Autodesk Inventor part; units mm, degrees
(part 4 of 4)
  arc A427 (4.3874, -10.8619) -> (4.7253, -10.6897) centre (-4.2393, 6.4866) ccw
  arc A428 (4.7253, -10.6897) -> (4.9404, -10.9173) centre (8.6621, -7.1833) ccw
  arc A429 (4.9404, -10.9173) -> (5.2279, -11.1867) centre (9.4643, -6.3793) ccw
  arc A430 (5.2279, -11.1867) -> (5.6027, -11.4963) centre (10.2445, -5.4945) ccw
  arc A431 (5.6027, -11.4963) -> (5.9512, -11.3011) centre (-4.2393, 6.4866) ccw
  arc A432 (5.9512, -11.3011) -> (5.8831, -10.8198) centre (-1.5915, -12.123) ccw
  arc A433 (5.8831, -10.8198) -> (5.8036, -10.4339) centre (-0.4294, -11.92) ccw
  arc A434 (5.8036, -10.4339) -> (5.7219, -10.1316) centre (0.6753, -11.6561) ccw
  arc A435 (5.7219, -10.1316) -> (6.0453, -9.9334) centre (-4.2393, 6.4866) ccw
  arc A436 (6.0453, -9.9334) -> (6.2776, -10.1434) centre (9.6948, -6.1289) ccw
  arc A437 (6.2776, -10.1434) -> (6.5853, -10.3895) centre (10.4315, -5.2644) ccw
  arc A438 (6.5853, -10.3895) -> (6.9833, -10.6687) centre (11.1399, -4.3212) ccw
  arc A439 (6.9833, -10.6687) -> (7.3154, -10.4467) centre (-4.2393, 6.4866) ccw
  arc A440 (7.3154, -10.4467) -> (7.2097, -9.9722) centre (-0.1395, -11.8579) ccw
  arc A441 (7.2097, -9.9722) -> (7.1002, -9.5938) centre (1.003, -11.5644) ccw
  arc A442 (7.1002, -9.5938) -> (6.9951, -9.2988) centre (2.0836, -11.2146) ccw
  arc A443 (6.9951, -9.2988) -> (7.3019, -9.0759) centre (-4.2393, 6.4866) ccw
  arc A444 (7.3019, -9.0759) -> (7.55, -9.267) centre (10.6417, -4.9968) ccw
  arc A445 (7.55, -9.267) -> (7.876, -9.4881) centre (11.3083, -4.0772) ccw
  arc A446 (7.876, -9.4881) -> (8.2947, -9.7353) centre (11.9405, -3.0813) ccw
  arc A447 (8.2947, -9.7353) -> (8.6084, -9.488) centre (-4.2393, 6.4866) ccw
  arc A448 (8.6084, -9.488) -> (8.4658, -9.0232) centre (1.2871, -11.4797) ccw
  arc A449 (8.4658, -9.0232) -> (8.3269, -8.6545) centre (2.4031, -11.0974) ccw
  arc A450 (8.3269, -8.6545) -> (8.199, -8.3687) centre (3.4529, -10.664) ccw
  arc A451 (8.199, -8.3687) -> (8.4873, -8.1224) centre (-4.2393, 6.4866) ccw
  arc A452 (8.4873, -8.1224) -> (8.7497, -8.2934) centre (11.4968, -3.7938) ccw
  arc A453 (8.7497, -8.2934) -> (9.0921, -8.4883) centre (12.0892, -2.8247) ccw
  arc A454 (9.0921, -8.4883) -> (9.5288, -8.7019) centre (12.6413, -1.7823) ccw
  arc A455 (9.5288, -8.7019) -> (9.8221, -8.4307) centre (-4.2393, 6.4866) ccw
  arc A456 (9.8221, -8.4307) -> (9.6435, -7.9786) centre (2.6797, -10.9907) ccw
  arc A457 (9.6435, -7.9786) -> (9.4761, -7.6219) centre (3.7622, -10.5221) ccw
  arc A458 (9.4761, -7.6219) -> (9.3261, -7.347) centre (4.7748, -10.0076) ccw
  arc A459 (9.3261, -7.347) -> (9.5943, -7.0788) centre (-4.2393, 6.4866) ccw
  arc A460 (9.5943, -7.0788) -> (9.8693, -7.2288) centre (12.2549, -2.5275) ccw
  arc A461 (9.8693, -7.2288) -> (10.2259, -7.3962) centre (12.7694, -1.5149) ccw
  arc A462 (10.2259, -7.3962) -> (10.678, -7.5748) centre (13.238, -0.4324) ccw
  arc A463 (10.678, -7.5748) -> (10.9492, -7.2815) centre (-4.2393, 6.4866) ccw
  arc A464 (10.9492, -7.2815) -> (10.7357, -6.8447) centre (4.0296, -10.394) ccw
  arc A465 (10.7357, -6.8447) -> (10.5408, -6.5023) centre (5.0721, -9.8418) ccw
  arc A466 (10.5408, -6.5023) -> (10.3697, -6.24) centre (6.0411, -9.2495) ccw
  arc A467 (10.3697, -6.24) -> (10.616, -5.9516) centre (-4.2393, 6.4866) ccw
  arc A468 (10.616, -5.9516) -> (10.9019, -6.0795) centre (12.9113, -1.2056) ccw
  arc A469 (10.9019, -6.0795) -> (11.2705, -6.2185) centre (13.3447, -0.1558) ccw
  arc A470 (11.2705, -6.2185) -> (11.7353, -6.3611) centre (13.727, 0.9602) ccw
  arc A471 (11.7353, -6.3611) -> (11.9826, -6.0473) centre (-4.2393, 6.4866) ccw
  arc A472 (11.9826, -6.0473) -> (11.7355, -5.6287) centre (5.3286, -9.6932) ccw
  arc A473 (11.7355, -5.6287) -> (11.5143, -5.3027) centre (6.3245, -9.0609) ccw
  arc A474 (11.5143, -5.3027) -> (11.3232, -5.0546) centre (7.2441, -8.3944) ccw
  arc A475 (11.3232, -5.0546) -> (11.5461, -4.7478) centre (-4.2393, 6.4866) ccw
  arc A476 (11.5461, -4.7478) -> (11.8411, -4.8528) centre (13.4619, 0.1637) ccw
  arc A477 (11.8411, -4.8528) -> (12.2196, -4.9624) centre (13.8117, 1.2443) ccw
  arc A478 (12.2196, -4.9624) -> (12.694, -5.0681) centre (14.1052, 2.3868) ccw
  arc A479 (12.694, -5.0681) -> (12.916, -4.736) centre (-4.2393, 6.4866) ccw
  arc A480 (12.916, -4.736) -> (12.6368, -4.338) centre (6.5685, -8.8926) ccw
  arc A481 (12.6368, -4.338) -> (12.3907, -4.0303) centre (7.5118, -8.1842) ccw
  arc A482 (12.3907, -4.0303) -> (12.1807, -3.798) centre (8.3762, -7.4475) ccw
  arc A483 (12.1807, -3.798) -> (12.3789, -3.4746) centre (-4.2393, 6.4866) ccw
  arc A484 (12.3789, -3.4746) -> (12.6812, -3.5562) centre (13.9035, 1.5721) ccw
  arc A485 (12.6812, -3.5562) -> (13.0671, -3.6358) centre (14.1674, 2.6768) ccw
  arc A486 (13.0671, -3.6358) -> (13.5484, -3.7039) centre (14.3703, 3.8388) ccw
  arc A487 (13.5484, -3.7039) -> (13.7436, -3.3554) centre (-4.2393, 6.4866) ccw
  arc A488 (13.7436, -3.3554) -> (13.434, -2.9806) centre (7.7419, -7.9972) ccw
  arc A489 (13.434, -2.9806) -> (13.1646, -2.6931) centre (8.6266, -7.217) ccw
  arc A490 (13.1646, -2.6931) -> (12.937, -2.478) centre (9.4306, -6.4148) ccw
  arc A491 (12.937, -2.478) -> (13.1092, -2.1401) centre (-4.2393, 6.4866) ccw
  arc A492 (13.1092, -2.1401) -> (13.417, -2.1977) centre (14.2331, 3.0107) ccw
  arc A493 (13.417, -2.1977) -> (13.8079, -2.2467) centre (14.4095, 4.1327) ccw
  arc A494 (13.8079, -2.2467) -> (14.2931, -2.2769) centre (14.5207, 5.307) ccw
  arc A495 (14.2931, -2.2769) -> (14.4604, -1.9141) centre (-4.2393, 6.4866) ccw
  arc A496 (14.4604, -1.9141) -> (14.1223, -1.5647) centre (8.8413, -7.0125) ccw
  arc A497 (14.1223, -1.5647) -> (13.8312, -1.2993) centre (9.6621, -6.1653) ccw
  arc A498 (13.8312, -1.2993) -> (13.5874, -1.1027) centre (10.4007, -5.3025) ccw
  arc A499 (13.5874, -1.1027) -> (13.7326, -0.7523) centre (-4.2393, 6.4866) ccw
  arc A500 (13.7326, -0.7523) -> (14.044, -0.7856) centre (14.4489, 4.4707) ccw
  arc A501 (14.044, -0.7856) -> (14.4375, -0.8038) centre (14.5367, 5.6031) ccw
  arc A502 (14.4375, -0.8038) -> (14.9236, -0.7958) centre (14.5554, 6.7826) ccw
  arc A503 (14.9236, -0.7958) -> (15.0618, -0.4211) centre (-4.2393, 6.4866) ccw
  arc A504 (15.0618, -0.4211) -> (14.6974, -0.0993) centre (9.8601, -5.9446) ccw
  arc A505 (14.6974, -0.0993) -> (14.3864, 0.1425) centre (10.6119, -5.0356) ccw
  arc A506 (14.3864, 0.1425) -> (14.1279, 0.3194) centre (11.2805, -4.1175) ccw
  arc A507 (14.1279, 0.3194) -> (14.2451, 0.6801) centre (-4.2393, 6.4866) ccw
  arc A508 (14.2451, 0.6801) -> (14.5582, 0.6713) centre (14.5494, 5.9432) ccw
  arc A509 (14.5582, 0.6713) -> (14.9519, 0.684) centre (14.5482, 7.079) ccw
  arc A510 (14.9519, 0.684) -> (15.4359, 0.7301) centre (14.4743, 8.2563) ccw
  arc A511 (15.4359, 0.7301) -> (15.5443, 1.1146) centre (-4.2393, 6.4866) ccw
  arc A512 (15.5443, 1.1146) -> (15.1558, 1.4068) centre (10.792, -4.8001) ccw
  arc A513 (15.1558, 1.4068) -> (14.8267, 1.6234) centre (11.4701, -3.8349) ccw
  arc A514 (14.8267, 1.6234) -> (14.5552, 1.7794) centre (12.0647, -2.8671) ccw
  arc A515 (14.5552, 1.7794) -> (14.6437, 2.1482) centre (-4.2393, 6.4866) ccw
  arc A516 (14.6437, 2.1482) -> (14.9565, 2.164) centre (14.5342, 7.419) ccw
  arc A517 (14.9565, 2.164) -> (15.3481, 2.2076) centre (14.4438, 8.5512) ccw
  arc A518 (15.3481, 2.2076) -> (15.8269, 2.2916) centre (14.2777, 9.7191) ccw
  arc A519 (15.8269, 2.2916) -> (15.9048, 2.6834) centre (-4.2393, 6.4866) ccw
  arc A520 (15.9048, 2.6834) -> (15.4946, 2.9442) centre (11.6312, -3.5859) ccw
  arc A521 (15.4946, 2.9442) -> (15.1495, 3.1343) centre (12.2315, -2.5705) ccw
  arc A522 (15.1495, 3.1343) -> (14.8666, 3.2686) centre (12.7483, -1.5591) ccw
  arc A523 (14.8666, 3.2686) -> (14.9259, 3.6431) centre (-4.2393, 6.4866) ccw
  arc A524 (14.9259, 3.6431) -> (15.2365, 3.6834) centre (14.4031, 8.8891) ccw
  arc A525 (15.2365, 3.6834) -> (15.6234, 3.7576) centre (14.2242, 10.0107) ccw
  arc A526 (15.6234, 3.7576) -> (16.0942, 3.8789) centre (13.967, 11.1619) ccw
  arc A527 (16.0942, 3.8789) -> (16.1411, 4.2756) centre (-4.2393, 6.4866) ccw
  arc A528 (16.1411, 4.2756) -> (15.7117, 4.5034) centre (12.3726, -2.3097) ccw
  arc A529 (15.7117, 4.5034) -> (15.3527, 4.6658) centre (12.8914, -1.2503) ccw
  arc A530 (15.3527, 4.6658) -> (15.0602, 4.7775) centre (13.3272, -0.2015) ccw
  arc A531 (15.0602, 4.7775) -> (15.0899, 5.1556) centre (-4.2393, 6.4866) ccw
  arc A532 (15.0899, 5.1556) -> (15.3964, 5.2201) centre (14.1572, 10.3443) ccw
  arc A533 (15.3964, 5.2201) -> (15.7763, 5.3244) centre (13.8908, 11.4485) ccw
  arc A534 (15.7763, 5.3244) -> (16.2361, 5.4823) centre (13.5441, 12.576) ccw
  arc A535 (16.2361, 5.4823) -> (16.2518, 5.8814) centre (-4.2393, 6.4866) ccw
  arc A536 (16.2518, 5.8814) -> (15.8058, 6.0748) centre (13.0115, -0.9792) ccw
  arc A537 (15.8058, 6.0748) -> (15.4352, 6.2086) centre (13.4456, 0.1176) ccw
  arc A538 (15.4352, 6.2086) -> (15.1348, 6.297) centre (13.7978, 1.1974) ccw
  arc A539 (15.1348, 6.297) -> (15.1348, 6.6762) centre (-4.2393, 6.4866) ccw
  arc A540 (15.1348, 6.6762) -> (15.4352, 6.7646) centre (13.7978, 11.7758) ccw
  arc A541 (15.4352, 6.7646) -> (15.8058, 6.8984) centre (13.4456, 12.8556) ccw
  arc A542 (15.8058, 6.8984) -> (16.2518, 7.0918) centre (13.0115, 13.9525) ccw
  arc A543 (16.2518, 7.0918) -> (16.2361, 7.491) centre (-4.2393, 6.4866) ccw
  arc A544 (16.2361, 7.491) -> (15.7763, 7.6488) centre (13.5441, 0.3973) ccw
  arc A545 (15.7763, 7.6488) -> (15.3964, 7.7531) centre (13.8908, 1.5248) ccw
  arc A546 (15.3964, 7.7531) -> (15.0899, 7.8177) centre (14.1572, 2.6289) ccw
  arc A547 (15.0899, 7.8177) -> (15.0602, 8.1957) centre (-4.2393, 6.4866) ccw
  arc A548 (15.0602, 8.1957) -> (15.3527, 8.3074) centre (13.3272, 13.1747) ccw
  arc A549 (15.3527, 8.3074) -> (15.7117, 8.4699) centre (12.8914, 14.2235) ccw
  arc A550 (15.7117, 8.4699) -> (16.1411, 8.6977) centre (12.3726, 15.2829) ccw
  arc A551 (16.1411, 8.6977) -> (16.0942, 9.0944) centre (-4.2393, 6.4866) ccw
  arc A552 (16.0942, 9.0944) -> (15.6234, 9.2156) centre (13.967, 1.8113) ccw
  arc A553 (15.6234, 9.2156) -> (15.2365, 9.2898) centre (14.2242, 2.9626) ccw
  arc A554 (15.2365, 9.2898) -> (14.9259, 9.3301) centre (14.4031, 4.0842) ccw
  arc A555 (14.9259, 9.3301) -> (14.8666, 9.7047) centre (-4.2393, 6.4866) ccw
  arc A556 (14.8666, 9.7047) -> (15.1495, 9.839) centre (12.7483, 14.5323) ccw
  arc A557 (15.1495, 9.839) -> (15.4946, 10.0291) centre (12.2315, 15.5438) ccw
  arc A558 (15.4946, 10.0291) -> (15.9048, 10.2899) centre (11.6312, 16.5592) ccw
  arc A559 (15.9048, 10.2899) -> (15.8269, 10.6817) centre (-4.2393, 6.4866) ccw
  arc A560 (15.8269, 10.6817) -> (15.3481, 10.7656) centre (14.2777, 3.2542) ccw
  arc A561 (15.3481, 10.7656) -> (14.9565, 10.8092) centre (14.4438, 4.422) ccw
  arc A562 (14.9565, 10.8092) -> (14.6437, 10.825) centre (14.5342, 5.5542) ccw
  arc A563 (14.6437, 10.825) -> (14.5552, 11.1938) centre (-4.2393, 6.4866) ccw
  arc A564 (14.5552, 11.1938) -> (14.8267, 11.3499) centre (12.0647, 15.8404) ccw
  arc A565 (14.8267, 11.3499) -> (15.1558, 11.5665) centre (11.4701, 16.8081) ccw
  arc A566 (15.1558, 11.5665) -> (15.5443, 11.8587) centre (10.792, 17.7733) ccw
  arc A567 (15.5443, 11.8587) -> (15.4359, 12.2431) centre (-4.2393, 6.4866) ccw
  arc A568 (15.4359, 12.2431) -> (14.9519, 12.2893) centre (14.4743, 4.717) ccw
  arc A569 (14.9519, 12.2893) -> (14.5582, 12.302) centre (14.5482, 5.8943) ccw
  arc A570 (14.5582, 12.302) -> (14.2451, 12.2932) centre (14.5494, 7.0301) ccw
  arc A571 (14.2451, 12.2932) -> (14.1279, 12.6539) centre (-4.2393, 6.4866) ccw
  arc A572 (14.1279, 12.6539) -> (14.3864, 12.8308) centre (11.2805, 17.0907) ccw
  arc A573 (14.3864, 12.8308) -> (14.6974, 13.0725) centre (10.6119, 18.0089) ccw
  arc A574 (14.6974, 13.0725) -> (15.0618, 13.3943) centre (9.8601, 18.9179) ccw
  arc A575 (15.0618, 13.3943) -> (14.9236, 13.7691) centre (-4.2393, 6.4866) ccw
  arc A576 (14.9236, 13.7691) -> (14.4375, 13.7771) centre (14.5554, 6.1907) ccw
  arc A577 (14.4375, 13.7771) -> (14.044, 13.7589) centre (14.5367, 7.3701) ccw
  arc A578 (14.044, 13.7589) -> (13.7326, 13.7256) centre (14.4489, 8.5025) ccw
  arc A579 (13.7326, 13.7256) -> (13.5874, 14.076) centre (-4.2393, 6.4866) ccw
  arc A580 (13.5874, 14.076) -> (13.8312, 14.2726) centre (10.4007, 18.2757) ccw
  arc A581 (13.8312, 14.2726) -> (14.1223, 14.538) centre (9.6621, 19.1385) ccw
  arc A582 (14.1223, 14.538) -> (14.4604, 14.8874) centre (8.8413, 19.9858) ccw
  arc A583 (14.4604, 14.8874) -> (14.2931, 15.2501) centre (-4.2393, 6.4866) ccw
  arc A584 (14.2931, 15.2501) -> (13.8079, 15.22) centre (14.5207, 7.6662) ccw
  arc A585 (13.8079, 15.22) -> (13.417, 15.171) centre (14.4095, 8.8406) ccw
  arc A586 (13.417, 15.171) -> (13.1092, 15.1133) centre (14.2331, 9.9626) ccw
  arc A587 (13.1092, 15.1133) -> (12.937, 15.4512) centre (-4.2393, 6.4866) ccw
  arc A588 (12.937, 15.4512) -> (13.1646, 15.6664) centre (9.4306, 19.388) ccw
  arc A589 (13.1646, 15.6664) -> (13.434, 15.9538) centre (8.6266, 20.1902) ccw
  arc A590 (13.434, 15.9538) -> (13.7436, 16.3286) centre (7.7419, 20.9705) ccw
  arc A591 (13.7436, 16.3286) -> (13.5484, 16.6771) centre (-4.2393, 6.4866) ccw
  arc A592 (13.5484, 16.6771) -> (13.0671, 16.609) centre (14.3703, 9.1345) ccw
  arc A593 (13.0671, 16.609) -> (12.6812, 16.5295) centre (14.1674, 10.2965) ccw
  arc A594 (12.6812, 16.5295) -> (12.3789, 16.4479) centre (13.9035, 11.4012) ccw
  arc A595 (12.3789, 16.4479) -> (12.1807, 16.7712) centre (-4.2393, 6.4866) ccw
  arc A596 (12.1807, 16.7712) -> (12.3907, 17.0036) centre (8.3762, 20.4208) ccw
  arc A597 (12.3907, 17.0036) -> (12.6368, 17.3113) centre (7.5118, 21.1574) ccw
  arc A598 (12.6368, 17.3113) -> (12.916, 17.7092) centre (6.5685, 21.8658) ccw
  arc A599 (12.916, 17.7092) -> (12.694, 18.0413) centre (-4.2393, 6.4866) ccw
  arc A600 (12.694, 18.0413) -> (12.2196, 17.9357) centre (14.1052, 10.5864) ccw
  arc A601 (12.2196, 17.9357) -> (11.8411, 17.8261) centre (13.8117, 11.7289) ccw
  arc A602 (11.8411, 17.8261) -> (11.5461, 17.721) centre (13.4619, 12.8095) ccw
  arc A603 (11.5461, 17.721) -> (11.3232, 18.0278) centre (-4.2393, 6.4866) ccw
  arc A604 (11.3232, 18.0278) -> (11.5143, 18.2759) centre (7.2441, 21.3676) ccw
  arc A605 (11.5143, 18.2759) -> (11.7355, 18.602) centre (6.3245, 22.0342) ccw
  arc A606 (11.7355, 18.602) -> (11.9826, 19.0206) centre (5.3286, 22.6664) ccw
  arc A607 (11.9826, 19.0206) -> (11.7353, 19.3343) centre (-4.2393, 6.4866) ccw
  arc A608 (11.7353, 19.3343) -> (11.2705, 19.1917) centre (13.727, 12.0131) ccw
  arc A609 (11.2705, 19.1917) -> (10.9019, 19.0528) centre (13.3447, 13.129) ccw
  arc A610 (10.9019, 19.0528) -> (10.616, 18.9249) centre (12.9113, 14.1788) ccw
  arc A611 (10.616, 18.9249) -> (10.3697, 19.2133) centre (-4.2393, 6.4866) ccw
  arc A612 (10.3697, 19.2133) -> (10.5408, 19.4756) centre (6.0411, 22.2227) ccw
  arc A613 (10.5408, 19.4756) -> (10.7357, 19.818) centre (5.0721, 22.8151) ccw
  arc A614 (10.7357, 19.818) -> (10.9492, 20.2547) centre (4.0296, 23.3672) ccw
  arc A615 (10.9492, 20.2547) -> (10.678, 20.548) centre (-4.2393, 6.4866) ccw
  arc A616 (10.678, 20.548) -> (10.2259, 20.3695) centre (13.238, 13.4056) ccw
  arc A617 (10.2259, 20.3695) -> (9.8693, 20.202) centre (12.7694, 14.4882) ccw
  arc A618 (9.8693, 20.202) -> (9.5943, 20.0521) centre (12.2549, 15.5007) ccw
  arc A619 (9.5943, 20.0521) -> (9.3261, 20.3202) centre (-4.2393, 6.4866) ccw
  arc A620 (9.3261, 20.3202) -> (9.4761, 20.5952) centre (4.7748, 22.9808) ccw
  arc A621 (9.4761, 20.5952) -> (9.6435, 20.9518) centre (3.7622, 23.4953) ccw
  arc A622 (9.6435, 20.9518) -> (9.8221, 21.4039) centre (2.6797, 23.964) ccw
  arc A623 (9.8221, 21.4039) -> (9.5288, 21.6751) centre (-4.2393, 6.4866) ccw
  arc A624 (9.5288, 21.6751) -> (9.0921, 21.4616) centre (12.6413, 14.7556) ccw
  arc A625 (9.0921, 21.4616) -> (8.7497, 21.2667) centre (12.0892, 15.798) ccw
  arc A626 (8.7497, 21.2667) -> (8.4873, 21.0956) centre (11.4968, 16.7671) ccw
  arc A627 (8.4873, 21.0956) -> (8.199, 21.3419) centre (-4.2393, 6.4866) ccw
  arc A628 (8.199, 21.3419) -> (8.3269, 21.6278) centre (3.4529, 23.6372) ccw
  arc A629 (8.3269, 21.6278) -> (8.4658, 21.9965) centre (2.4031, 24.0707) ccw
  arc A630 (8.4658, 21.9965) -> (8.6084, 22.4612) centre (1.2871, 24.4529) ccw
  arc A631 (8.6084, 22.4612) -> (8.2947, 22.7085) centre (-4.2393, 6.4866) ccw
  arc A632 (8.2947, 22.7085) -> (7.876, 22.4614) centre (11.9405, 16.0545) ccw
  arc A633 (7.876, 22.4614) -> (7.55, 22.2402) centre (11.3083, 17.0504) ccw
  arc A634 (7.55, 22.2402) -> (7.3019, 22.0491) centre (10.6417, 17.97) ccw
  arc A635 (7.3019, 22.0491) -> (6.9951, 22.272) centre (-4.2393, 6.4866) ccw
  arc A636 (6.9951, 22.272) -> (7.1002, 22.567) centre (2.0836, 24.1879) ccw
  arc A637 (7.1002, 22.567) -> (7.2097, 22.9455) centre (1.003, 24.5376) ccw
  arc A638 (7.2097, 22.9455) -> (7.3154, 23.42) centre (-0.1395, 24.8311) ccw
  arc A639 (7.3154, 23.42) -> (6.9833, 23.6419) centre (-4.2393, 6.4866) ccw
  circle A640 centre (-4.2393, 6.4866) radius 2
  circle A641 centre (-4.2393, 6.4866) radius 18.25
  point P0 (0, 0)
  dimension "d31" = 36.5
  constraints: 1 centre point, 1 coincident
  measures "d31" diameter of A641
extrude "押し出し9" cut sketch "スケッチ3" against normal blind 0.75 contours A641
sketch "スケッチ4" plane through (4.2393, 6.4866, 2.25) normal (0, 0, 1) x (1, 0, 0)
  circle A0 centre (0, 0) radius 18.25
  circle A1 centre (0, 0) radius 2
  circle A2 centre (0, 0) radius 16.25
  circle A3 centre (0, 0) radius 6
  line L0 (0, 2) -> (0, 16.25) construction
  line L1 (1.9988, 2.0702) -> (1.4991, 16.3026)
  line L2 (-1.4991, 16.3026) -> (-1.9988, 2.0702)
  arc A4 (-1.9988, 2.0702) -> (1.9988, 2.0702) centre (0, 2) ccw
  arc A5 (1.4991, 16.3026) -> (-1.4991, 16.3026) centre (0, 16.25) ccw
  line L3 (-16.3026, -1.4991) -> (-2.0702, -1.9988)
  line L4 (-2.0702, 1.9988) -> (-16.3026, 1.4991)
  line L5 (1.4991, -16.3026) -> (1.9988, -2.0702)
  line L6 (-1.9988, -2.0702) -> (-1.4991, -16.3026)
  line L7 (16.3026, 1.4991) -> (2.0702, 1.9988)
  line L8 (2.0702, -1.9988) -> (16.3026, -1.4991)
  point P0 (-4.2393, -6.4866)
  point P1 (0, 9.125)
  point P2 (5.7007, 1.8713)
  point P3 (16.1803, 1.5034)
  point P4 (1.5034, 16.1803)
  point P5 (1.8713, 5.7007)
  point P6 (16.1803, -1.5034)
  point P7 (5.7007, -1.8713)
  point P8 (1.8713, -5.7007)
  point P9 (1.5034, -16.1803)
  point P10 (-1.5034, -16.1803)
  point P11 (-1.8713, -5.7007)
  point P12 (-5.7007, -1.8713)
  point P13 (-16.1803, -1.5034)
  point P14 (-16.1803, 1.5034)
  point P15 (-5.7007, 1.8713)
  point P16 (-1.8713, 5.7007)
  point P17 (-1.5034, 16.1803)
  dimension "d34" = 2
  dimension "d35" = 12
  dimension "d36" = 3
  dimension "d39" = 360
  dimension "d44" = 2
  constraints: 20 end point, 4 point on circle, 4 tangent, 3 centre point, 2 vertical, 1 coincident, 1 midpoint, 1 vertical alignment, 29 other
  measures "d35" diameter of A3
  measures "d36" diameter of A5
  measures "d44" radius of A4
extrude "押し出し10" cut sketch "スケッチ4" against normal blind 3 contours L1 A2 L7 A3 | A3 L4 A2 L2 | A3 L6 A2 L3 | L8 A2 L5 A3
fillet "フィレット1" radius 1.05 16 edges at (-11.941, 7.99, 1.5) (2.368, 12.1873, 1.5) (-1.4614, 8.3579, 1.5) (2.7359, 22.6669, 1.5) (-1.4614, 4.6153, 1.5) (2.368, 0.7859, 1.5) (-11.941, 4.9833, 1.5) (5.7427, 22.6669, 1.5) (2.7359, -9.6937, 1.5) (20.4196, 7.99, 1.5) (9.94, 8.3579, 1.5) (6.1106, 12.1873, 1.5) (5.7427, -9.6937, 1.5) (6.1106, 0.7859, 1.5) (9.94, 4.6153, 1.5) (20.4196, 4.9833, 1.5)
sketch "スケッチ6" plane through (4.2393, 6.4866, 0.75) normal (0, 0, -1) x (-1, 0, 0)
  circle A0 centre (0, 0) radius 2
  circle A1 centre (0, 0) radius 2
  circle A2 centre (0, 0) radius 6
  point P0 (4.2393, -6.4866)
  dimension "d49" = 4
  dimension "d50" = 12
  constraints: 2 centre point, 2 coincident
  measures "d49" diameter of A1
  measures "d50" diameter of A2
extrude "押し出し12" add sketch "スケッチ6" along normal blind 0.75
